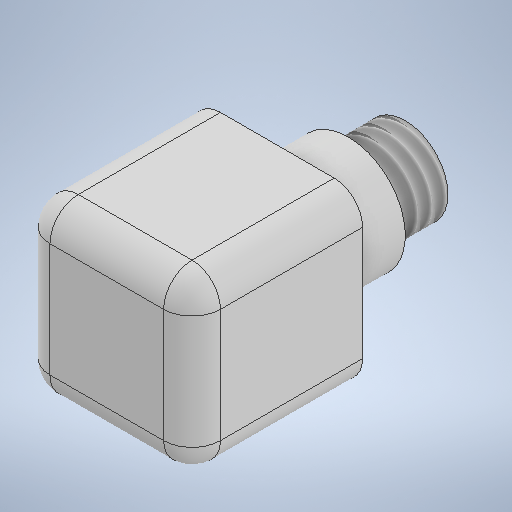
# Autodesk Inventor part: CONECTOR L-F
Saved by Autodesk Inventor 2025.2 (Build 292293000, 293)
## iProperties
Created: 2025-05-14
Part Number: CONECTOR L-F
Material: Genérico
Document SubType Name: Modeling
Designer: marce
Density: 1 g/cm^3
Appearance: Padrão
Author: marce
Autodesk Inventor part; units mm, degrees
ref_plane "YZ Plane" through (0, 0, 0) normal (1, 0, 0) x (0, 1, 0)
ref_plane "XZ Plane" through (0, 0, 0) normal (0, 1, 0) x (-1, 0, 0)
ref_plane "XY Plane" through (0, 0, 0) normal (0, 0, 1) x (1, 0, 0)
sketch "Esboço1" plane through (0, 0, 0) normal (1, 0, 0) x (0, 1, 0)
  line L0 (0, 0) -> (6, 0)
  line L1 (6, 0) -> (6, -6)
  line L2 (6, -6) -> (0, -6)
  line L3 (0, -6) -> (0, 0)
  dimension "d0" = 6
  dimension "d1" = 6
  constraints: 8 end point, 2 parallel, 1 horizontal, 1 perpendicular
  measures "d0" distance of L1.end L2.end
  measures "d1" distance of L0.end L1.end
extrude "Extrusão1" add sketch "Esboço1" along normal blind 6
sketch "Esboço2" plane through (0, 0, -6) normal (0, -1, 0) x (1, 0, 0)
  line L0 (0, 6) -> (6, 6) projected
  line L1 (0, 0) -> (6, 0) projected
  point P0 (3, 3)
hole "Furo1" at (3, 0, -3) direction (0, 1, 0) diameter 3.242 depth 4 thread size "M4x0.7" class "6H" standard "ANSI Metric M Profile"
sketch "Esboço3" plane through (0, 0, -6) normal (0, 0, -1) x (-1, 0, 0)
  line L0 (0, 0) -> (-6, 0) projected
  line L1 (0, 6) -> (-6, 6) projected
  circle A0 centre (-3, 3) radius 2
  dimension "d11" = 4
  constraints: 1 centre point, 1 coincident
  measures "d11" diameter of A0
extrude "Extrusão2" add sketch "Esboço3" along normal blind 2.5
sketch "Esboço4" plane through (3, 3, -8.5) normal (0, 0, -1) x (-1, 0, 0)
  point P0 (3, -3)
  point P1 (0, 0)
sketch "Esboço7" plane through (3, 3, -8.5) normal (0, 0, -1) x (-1, 0, 0)
  circle A0 centre (0, 0) radius 1.5
  point P0 (3, -3)
  dimension "d20" = 3
  constraints: 1 centre point
  measures "d20" diameter of A0
extrude "Extrusão4" add sketch "Esboço7" along normal blind 2
thread "Rosca2" size "M3x0.5" class "6g" standard "ANSI Metric M Profile" full length
fillet "Arredondamento1" radius 1 1 edges at (6, 0, -3)
fillet "Arredondamento2" radius 1 3 edges at (6, 3.5, 0) (5.7071, 0.2929, 0) (2.5, 0, 0)
fillet "Arredondamento3" radius 1 3 edges at (0, 3.5, 0) (0, 0.2929, -0.2929) (0, 0, -3.5)
fillet "Arredondamento4" radius 1 5 edges at (3, 6, 0) (5.7071, 6, -0.2929) (6, 6, -3.5) (0.2929, 6, -0.2929) (0, 6, -3.5)
